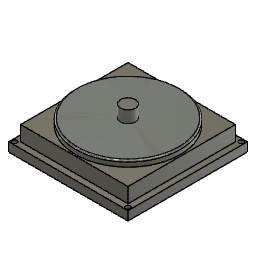
Peça 1 v3 (Autodesk Fusion 360 design; units mm, degrees)
Autodesk Fusion 360 part; units mm, degrees
sketch "Sketch1" plane through (0, 0, 0) normal (0, 1, 0) x (1, 0, 0)
  line L0 (90, -90) -> (-90, -90)
  line L1 (-90, -90) -> (-90, 90)
  line L2 (-90, 90) -> (90, 90)
  line L3 (90, 90) -> (90, -90)
  line L4 (90, -90) -> (-90, 90) construction
  line L5 (-90, -90) -> (90, 90) construction
  line L6 (100, -100) -> (-100, -100)
  line L7 (-100, -100) -> (-100, 100)
  line L8 (-100, 100) -> (100, 100)
  line L9 (100, 100) -> (100, -100)
  line L10 (100, -100) -> (-100, 100) construction
  line L11 (-100, -100) -> (100, 100) construction
  line L12 (-100, 100) -> (-90, 90)
  line L13 (100, 100) -> (90, 90)
  line L14 (90, -90) -> (100, -100)
  line L15 (-90, -90) -> (-100, -100)
  circle A0 centre (-95, -95) radius 4
  circle A1 centre (-95, 95) radius 4
  circle A2 centre (95, 95) radius 4
  circle A3 centre (95, -95) radius 4
  dimension "d3" = 180
  dimension "d4" = 180
  dimension "d5" = 200
  dimension "d6" = 200
  dimension "d7" = 8
  dimension "d8" = 8
  dimension "d9" = 8
  dimension "d10" = 8
  constraint horizontal L0
  constraint perpendicular L0 L1
  constraint parallel L0 L2
  constraint parallel L1 L3
  constraint coincident L4 origin
  constraint coincident L5 origin
  constraint horizontal L6
  constraint perpendicular L6 L7
  constraint parallel L6 L8
  constraint parallel L7 L9
  constraint coincident L10 origin
  constraint coincident L11 origin
  constraint midpoint L15 A0.centre
  constraint midpoint L12 A1.centre
  constraint midpoint L13 A2.centre
  constraint midpoint L14 A3.centre
  measures "d3" distance of L1.end L2.end
  measures "d4" distance of L0.end L1.end
  measures "d5" distance of L7.end L8.end
  measures "d6" distance of L6.end L7.end
  measures "d7" diameter of A0
  measures "d8" diameter of A1
  measures "d9" diameter of A2
  measures "d10" diameter of A3
extrude "Extrude1" add sketch "Sketch1" along normal blind 40 contours L0 L1 L2 L3
extrude "Extrude2" add sketch "Sketch1" along normal blind 15 contours L0 L6 L14 L15 A0 A3 | L3 L9 L13 L14 A2 A3 | L1 L7 L12 L15 A0 A1 | L2 L8 L12 L13 A1 A2
sketch "Sketch2" plane through (0, 40, 0) normal (0, 1, 0) x (-1, 0, 0)
  line L0 (-90, -90) -> (90, -90)
  line L1 (90, -90) -> (90, 90)
  line L2 (90, 90) -> (-90, 90)
  line L3 (-90, 90) -> (-90, -90)
  circle A0 centre (0, 0) radius 87.5
  circle A1 centre (0, 0) radius 12.5
  dimension "d15" = 175
  dimension "d16" = 25
  constraint coincident A0.centre A1.centre
  constraint concentric A0 A1
  measures "d15" diameter of A0
  measures "d16" diameter of A1
extrude "Extrude3" add sketch "Sketch2" along normal blind 30 contours A1
extrude "Extrude4" add sketch "Sketch2" along normal blind 10 contours A0
fillet "Fillet1" radius 2.5 1 edges at (81.5786, 50, -31.6414)
sketch "Sketch3" plane through (0, 50, 0) normal (0, 1, 0) x (-1, 0, 0)
  circle A0 centre (0, 0) radius 12.5
  circle A1 centre (0, 0) radius 85
